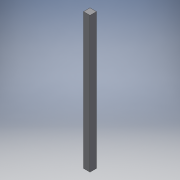
# Autodesk Inventor part: square shaft 1
Saved by Autodesk Inventor 2017 (Build 210142000, 142)
## iProperties
Created: 2018-04-16
Part Number: square shaft 1
Material: Generic
Document SubType Name: Modeling
Designer: RKL
Density: 1 g/cm^3
Appearance: Default
Author: RKL
Autodesk Inventor part; units mm, degrees
ref_plane "YZ Plane" through (0, 0, 0) normal (1, 0, 0) x (0, 1, 0)
ref_plane "XZ Plane" through (0, 0, 0) normal (0, 1, 0) x (-1, 0, 0)
ref_plane "XY Plane" through (0, 0, 0) normal (0, 0, 1) x (1, 0, 0)
sketch "Sketch1" plane through (0, 0, 0) normal (0, 0, 1) x (1, 0, 0)
  line L0 (4.7625, -4.7625) -> (-4.7625, -4.7625)
  line L1 (-4.7625, -4.7625) -> (-4.7625, 4.7625)
  line L2 (-4.7625, 4.7625) -> (4.7625, 4.7625)
  line L3 (4.7625, 4.7625) -> (4.7625, -4.7625)
  line L4 (4.7625, -4.7625) -> (-4.7625, 4.7625) construction
  line L5 (-4.7625, -4.7625) -> (4.7625, 4.7625) construction
  point P0 (0, 0)
  dimension "d0" = 9.525
  constraints: 12 end point, 2 midpoint, 2 parallel, 2 perpendicular, 1 horizontal
  measures "d0" distance of L0.end L1.end
extrude "Extrusion1" add sketch "Sketch1" along normal blind 200
body "Solid1"
